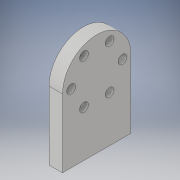
# Autodesk Inventor part: thumb mount
Saved by Autodesk Inventor 2018 (Build 220112000, 112)
## iProperties
Created: 2020-04-07
Part Number: thumb mount
Material: Generic
Document SubType Name: Modeling
Designer: Jesse R-B
Density: 1 g/cm^3
Appearance: Default
Author: Jesse R-B
Autodesk Inventor part; units mm, degrees
ref_plane "YZ Plane" through (0, 0, 0) normal (1, 0, 0) x (0, 1, 0)
sketch "Sketch1" plane through (0, 0, 0) normal (1, 0, 0) x (0, 1, 0)
  circle A0 centre (0, 0) radius 12.7
  circle A1 centre (0, 0) radius 6
  circle A2 centre (0, 9.525) radius 1.63
  circle A3 centre (8.2489, 4.7625) radius 1.63
  circle A4 centre (8.2489, -4.7625) radius 1.63
  circle A5 centre (0, -9.525) radius 1.63
  circle A6 centre (-8.2489, -4.7625) radius 1.63
  circle A7 centre (-8.2489, 4.7625) radius 1.63
  circle A8 centre (0, 0) radius 6
  circle A9 centre (0, 0) radius 3.2
  point P0 (0, 0.0001)
  constraints: 10 centre point
extrude "Extrusion1" add sketch "Sketch1" along normal blind 5.0038 contours A0 | A1 | A9
sketch "Sketch2" plane through (0, 0, 0) normal (-1, 0, 0) x (0, 0, 1)
  circle A0 centre (0, 0) radius 12.7 projected
  line L0 (12.7, 0) -> (12.7, -25.4)
  line L1 (0, 0) -> (0, -12.7) construction
  line L2 (-12.7, 0) -> (-12.7, -25.4)
  line L3 (12.7, -25.4) -> (-12.7, -25.4)
  circle A1 centre (-9.525, 0) radius 1.63 projected
  circle A2 centre (-4.7625, 8.2489) radius 1.63 projected
  circle A3 centre (4.7625, 8.2489) radius 1.63 projected
  circle A4 centre (4.7625, -8.2489) radius 1.63 projected
  circle A5 centre (-4.7625, -8.2489) radius 1.63 projected
  circle A6 centre (9.525, 0) radius 1.63 projected
  circle A7 centre (0, 0) radius 12.7 projected
  arc A8 (-12.7, 0) -> (12.7, 0) centre (0, 0) ccw
  dimension "d2" = 25.4
  constraints: 8 end point, 5 point on circle, 2 symmetric about line, 2 tangent, 2 vertical, 1 centre point, 1 horizontal
  measures "d2" distance of L0.start L0.end
extrude "Extrusion2" add sketch "Sketch2" against normal blind 5.0038 contours L0 L3 L2 A0
ref_plane "Work Plane1" through (2.5019, 0, 0) normal (-1, 0, 0) x (0, 0, 1)
ref_plane "Work Plane2" through (0, -25.4, 0) normal (0, 0, -1) x (-1, 0, 0)
body "Solid1"
